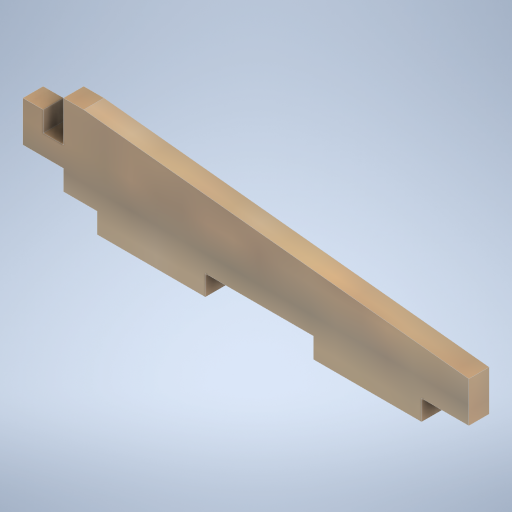
# Autodesk Inventor part: tail fin
Saved by Autodesk Inventor 2023 (Build 270158000, 158)
## iProperties
Created: 2023-06-06
Part Number: tail fin
Material: Hardboard
Document SubType Name: Sheet Metal
Designer: Ronan
Density: 0.799949 g/cm^3
Sheet Metal Rule: Default_mm
Appearance: Natural Maple - Glossy Dark Tint(1)
Author: Ronan
Autodesk Inventor part; units mm, degrees
ref_plane "YZ Plane" through (0, 0, 0) normal (1, 0, 0) x (0, 1, 0)
ref_plane "XZ Plane" through (0, 0, 0) normal (0, 1, 0) x (-1, 0, 0)
ref_plane "XY Plane" through (0, 0, 0) normal (0, 0, 1) x (1, 0, 0)
sketch "Sketch1" plane through (0, 0, 0) normal (0, 0, 1) x (1, 0, 0)
  line L0 (0, 0) -> (0, 12)
  line L1 (60, 6) -> (60, 0)
  line L2 (60, 0) -> (0, 0)
  line L3 (0, 3) -> (-6, 3)
  line L4 (-6, 3) -> (-6, 9)
  line L5 (-6, 9) -> (-3, 9)
  line L6 (-3, 9) -> (-3, 6)
  line L7 (-3, 6) -> (0, 6)
  line L8 (5, 0) -> (21, 0)
  line L9 (21, 0) -> (21, -3)
  line L10 (21, -3) -> (5, -3)
  line L11 (5, -3) -> (5, 0)
  line L12 (37, 0) -> (53, 0)
  line L13 (53, 0) -> (53, -3)
  line L14 (53, -3) -> (37, -3)
  line L15 (37, -3) -> (37, 0)
  line L16 (0, 12) -> (3, 12)
  line L17 (3, 12) -> (60, 6)
  dimension "d0" = 3
  dimension "d1" = 3
  dimension "d2" = 3
  dimension "d3" = 3
  dimension "d4" = 3
  dimension "d5" = 3
  dimension "d6" = 16
  dimension "d7" = 5
  dimension "d8" = 16
  dimension "d9" = 7
  dimension "d10" = 3
  dimension "d11" = 6
  dimension "d12" = 3
  constraints: 36 end point, 6 perpendicular, 5 parallel, 4 horizontal, 3 point on line, 2 equal length, 1 midpoint, 1 vertical
  measures "d0" distance between parallel lines of L2 L3
  measures "d1" distance between parallel lines of L3 L7
  measures "d2" distance between parallel lines of L7 L5
  measures "d3" distance between parallel lines of L0 L6
  measures "d4" distance of L4.end L5.end
  measures "d5" distance of L10.end L8.start
  measures "d6" distance of L13.end L14.end
  measures "d7" distance between parallel lines of L11 L0
  measures "d8" distance between parallel lines of L15 L9
  measures "d9" distance between parallel lines of L13 L1
  measures "d10" distance from line of L0.end L5
  measures "d11" distance of L1.start L1.end
  measures "d12" distance of L0.end L16.end
extrude "Extrusion1" add sketch "Sketch1" along normal blind 3
equation "\"BendRadius\" = Thickness"
equation "\"BendReliefWidth\" = Thickness"
equation "\"BendReliefDepth\" = 0.5 * Thickness"
equation "\"CornerReliefSize\" = 4 * Thickness"
equation "\"MinimumRemnant\" = 2 * Thickness"
equation "\"TransitionRadius\" = BendRadius"
equation "\"JacobiRadiusSize\" = BendRadius"
equation "\"GapSize\" = Thickness"
equation "\"Thickness\" = 0.5"
body "Solid1"
